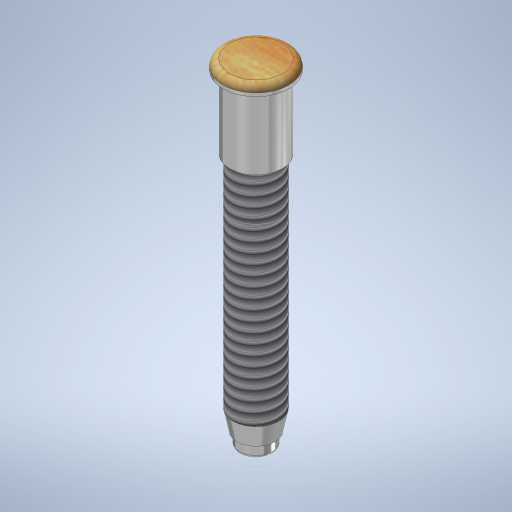
# Autodesk Inventor part: Confirmat L50 & Cap D10 NB T18 PB T 18
Saved by Autodesk Inventor 2024 (Build 280153000, 153)
## iProperties
Created: 2009-08-21
Part Number: Confirmat L50 & Cap D10 NB T18 PB T 18
Material: Nickel-Copper Alloy 400
Description: Confirmat & Cap
Document SubType Name: Modeling
Designer: Saulius Dereskeviciu
Mass: 24.4108 g
Surface Area: 16.8956 cm^2
Volume: 2.76453 cm^3
Density: 8.83 g/cm^3
Appearance: Chrome - Polished
Perskaiciuoti: 1
Author: Saulius Dereskeviciu
Autodesk Inventor part; units mm, degrees
ref_plane "YZ Plane" through (0, 0, 0) normal (1, 0, 0) x (0, 1, 0)
ref_plane "XZ Plane" through (0, 0, 0) normal (0, 1, 0) x (-1, 0, 0)
ref_plane "XY Plane" through (0, 0, 0) normal (0, 0, 1) x (1, 0, 0)
sketch "Sketch2" plane through (0, 0, 0) normal (1, 0, 0) x (0, 1, 0)
  line L0 (0, 0) -> (-5, 0)
  line L1 (-5, -0.5) -> (-4, -1)
  line L2 (-3.5, -12) -> (-3.5, -45)
  line L3 (-3.5, -45) -> (-2.9, -48)
  line L4 (0, -50) -> (0, 0)
  line L5 (-5, -0.5) -> (-5, 0)
  line L6 (-2.5, -50) -> (0, -50)
  line L7 (-2.5, -50) -> (-2.5, -48)
  line L8 (-2.5, -48) -> (-2.9, -48)
  line L9 (-4, -1) -> (-4, -11.5)
  line L10 (-3.5, -12) -> (-4, -11.5)
  dimension "d0" = 10
  dimension "d1" = 5
  dimension "d2" = 7
  dimension "d3" = 3
  dimension "d4" = 2
  dimension "d5" = 0.6
  dimension "Length" = 50
  dimension "d7" = 8
  dimension "d9" = 0.5
  dimension "d10" = 1
  dimension "d17" = 12
  dimension "d18" = 135
  constraints: 22 end point, 7 perpendicular, 1 horizontal
  measures "d0" diameter of L5 L4
  measures "d1" diameter of L7 L4
  measures "d2" diameter of L2 L4
  measures "d3" vertical distance of L2.end L3.end
  measures "d4" distance of L6.start L7.end
  measures "d5" distance from line of L3.end L2
  measures "Length" distance between parallel lines of L6 L0
  measures "d7" diameter of L9 L4
  measures "d9" distance of L1.start L0.end
  measures "d10" distance from line of L0 L1.end
  measures "d17" distance from line of L0 L2.start
  measures "d18" angle of L9 L10
revolve "Revolution1" add sketch "Sketch2" angle 360 about axis through (0, 0, -50) along (0, 0, 1)
thread "Thread1" size "TR8x1.5" class "7e" standard "ISO Metric Trapezoidal Threads" full length
sketch "Sketch3" plane through (0, 0, 0) normal (0, 0, 1) x (1, 0, 0)
  circle A0 centre (0, 0) radius 5 projected
  circle A1 centre (0, 0) radius 2.5 construction
  line L0 (1.4434, 2.5) -> (2.8868, 0)
  line L1 (2.8868, 0) -> (1.4434, -2.5)
  line L2 (1.4434, -2.5) -> (-1.4434, -2.5)
  line L3 (-1.4434, -2.5) -> (-2.8868, 0)
  line L4 (-2.8868, 0) -> (-1.4434, 2.5)
  line L5 (-1.4434, 2.5) -> (1.4434, 2.5)
  point P0 (0, 2.5)
  dimension "d14" = 5
  constraints: 12 end point, 2 coincident, 1 midpoint, 1 vertical alignment, 15 other
extrude "Extrusion1" cut sketch "Sketch3" against normal blind 4 draft -5 contours L0 L1 L2 L3 L4 L5
fillet "Fillet1" radius 0.5 1 edges at (0, 2.5, -50)
sketch "Sketch4" plane through (0, 0, 0) normal (0, 0, 1) x (1, 0, 0)
  circle A0 centre (0, 0) radius 5 construction
  circle A1 centre (0, 0) radius 4
  dimension "d20" = 8
  constraints: 1 centre point, 1 coincident
  measures "d20" diameter of A1
extrude "Extrusion2" add sketch "Sketch4" against normal blind 18 separate body
sketch "Sketch5" plane through (0, 0, -18) normal (0, 0, -1) x (-1, 0, 0)
  circle A0 centre (0, 0) radius 4 projected
  circle A1 centre (0, 0) radius 2.5
  dimension "d23" = 5
  constraints: 1 centre point, 1 coincident
  measures "d23" diameter of A1
extrude "Extrusion3" add sketch "Sketch5" along normal blind 33 contours A1 bodies 2
sketch "Sketch6" plane through (0, 0, 0) normal (0, 1, 0) x (-1, 0, 0)
  line L0 (0, 0) -> (-5, 0)
  line L1 (-5, 0) -> (-5, 1)
  line L2 (-5, 1) -> (0, 1)
  line L3 (0, 1) -> (0, 0)
  dimension "d26" = 10
  dimension "d27" = 1
  constraints: 8 end point, 2 parallel, 1 horizontal, 1 perpendicular
  measures "d26" diameter of L1 L3
  measures "d27" distance of L0.end L1.end
revolve "Revolution2" add sketch "Sketch6" angle 360 about axis through (0, 0, 1) along (0, 0, -1) separate body
fillet "Fillet2" radius 1 1 edges at (-5, 0, 1)
equation "\"Pillar_Board_Thickness\" = 18"
equation "\"d31\" = -0.5 * Pillar_Board_Thickness"
